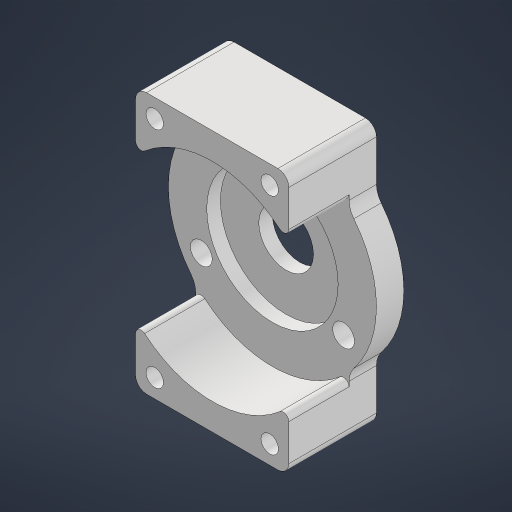
# Autodesk Inventor part: MotorMount_sub
Saved by Autodesk Inventor 2024.2 (Build 282272000, 272)
## iProperties
Created: 2023-12-20
Part Number: MotorMount_sub
Material: 一般
Document SubType Name: Modeling
Designer: Hanaoka
Density: 1 g/cm^3
Appearance: 既定
Author: Hanaoka
Autodesk Inventor part; units mm, degrees
ref_plane "YZ Plane" through (0, 0, 0) normal (1, 0, 0) x (0, 1, 0)
ref_plane "XZ Plane" through (0, 0, 0) normal (0, 1, 0) x (-1, 0, 0)
ref_plane "XY Plane" through (0, 0, 0) normal (0, 0, 1) x (1, 0, 0)
sketch "スケッチ1" plane through (0, 0, 0) normal (0, 0, 1) x (1, 0, 0)
  circle A0 centre (0, 0) radius 2.5
  circle A1 centre (0, 0) radius 6
  circle A2 centre (0, 0) radius 9.5
  circle A3 centre (0, 7.5) radius 1
  circle A4 centre (0, 0) radius 7.5 construction
  line L0 (0, -20.3) -> (0, 20.3) projected
  circle A5 centre (-6.4952, -3.75) radius 1
  circle A6 centre (6.4952, -3.75) radius 1
  circle A7 centre (0, 0) radius 14.5 construction
  line L1 (-7, 6.4226) -> (-7, 10.9226)
  line L2 (-6, 11.9226) -> (6, 11.9226)
  line L3 (7, 10.9226) -> (7, 6.4226)
  arc A8 (-6, 11.9226) -> (-7, 10.9226) centre (-6, 10.9226) ccw
  arc A9 (7, 10.9226) -> (6, 11.9226) centre (6, 10.9226) ccw
  circle A10 centre (5.25, 10.2317) radius 2 construction
  circle A11 centre (5.25, 10.2317) radius 0.8
  circle A12 centre (-5.25, 10.2317) radius 2 construction
  circle A13 centre (-5.25, 10.2317) radius 0.8
  line L4 (-5.25, 10.2317) -> (-5.25, 7.9175) construction
  line L5 (5.25, 10.2317) -> (5.25, 7.9175) construction
  circle A14 centre (5.25, -10.2317) radius 0.8
  line L6 (7, -6.4226) -> (7, -10.9226)
  arc A15 (6, -11.9226) -> (7, -10.9226) centre (6, -10.9226) ccw
  line L7 (6, -11.9226) -> (-6, -11.9226)
  circle A16 centre (-5.25, -10.2317) radius 2 construction
  line L8 (-7, -10.9226) -> (-7, -6.4226)
  arc A17 (-7, -10.9226) -> (-6, -11.9226) centre (-6, -10.9226) ccw
  circle A18 centre (-5.25, -10.2317) radius 0.8
  circle A19 centre (5.25, -10.2317) radius 2 construction
  dimension "d4" = 15
  dimension "d0" = 5
  dimension "d1" = 12
  dimension "d2" = 19
  dimension "d3" = 2
  dimension "d7" = 360
  dimension "d13" = 29
  dimension "d14" = 1
  dimension "d15" = 12
  dimension "d16" = 4.5
  dimension "d17" = 4
  dimension "d18" = 1.6
  dimension "d19" = 10.5
  dimension "d22" = 360
  constraints: 19 centre point, 16 end point, 12 point on circle, 9 coincident, 5 tangent, 3 equal radius, 3 parallel, 2 perpendicular, 2 vertical, 1 horizontal alignment, 1 point on line, 1 vertical alignment, 52 other
  measures "d0" diameter of A0
  measures "d1" diameter of A1
  measures "d2" diameter of A2
  measures "d3" diameter of A3
  measures "d13" diameter of A7
  measures "d14" radius of A8
  measures "d15" distance of L2.start L2.end
  measures "d16" distance of L3.start L3.end
  measures "d17" diameter of A10
  measures "d18" diameter of A11
  measures "d19" distance between parallel lines of L4 L5
extrude "押し出し1" add sketch "スケッチ1" along normal blind 1.25 contours A0 L0 A1 | A0 L0 A1 | L0 A3 A2 A1 | A1 L0 A2 A3
extrude "押し出し2" add sketch "スケッチ1" along normal blind 2.5 contours L0 A3 A2 A1 | A1 L0 A2 A3
extrude "押し出し3" add sketch "スケッチ1" along normal blind 8 contours L0 L7 A17 L8 A2 | A2 L6 A15 L7 L0 | L0 L2 A9 L3 A2 | A2 L1 A8 L2 L0
fillet "フィレット1" radius 2 4 edges at (-7, 6.4226, 1.25) (-7, -6.4226, 1.25) (7, 6.4226, 1.25) (7, -6.4226, 1.25)
fillet "フィレット2" radius 0.5 4 edges at (7, 6.4226, 5.25) (7, -6.4226, 5.25) (-7, -6.4226, 5.25) (-7, 6.4226, 5.25)
